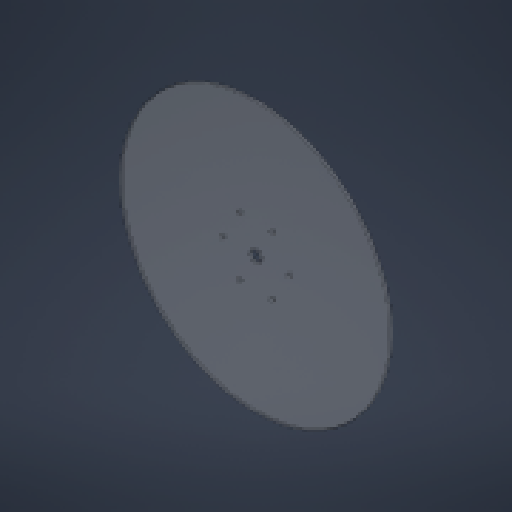
# Autodesk Inventor part: PLATE,BOTTOM
Saved by Autodesk Inventor 2026 (Build 300175000, 175)
## iProperties
Created: 2026-02-06
Part Number: PLATE,BOTTOM
Material: Polycarbonate, Clear
Document SubType Name: Sheet Metal
Designer: littl
Density: 1.2 g/cm^3
Sheet Metal Rule: Default
Appearance: Polycarbonate - Clear
Author: littl
Autodesk Inventor part; units mm, degrees
ref_plane "YZ Plane" through (0, 0, 0) normal (1, 0, 0) x (0, 1, 0)
ref_plane "XZ Plane" through (0, 0, 0) normal (0, 1, 0) x (-1, 0, 0)
ref_plane "XY Plane" through (0, 0, 0) normal (0, 0, 1) x (1, 0, 0)
sketch "Sketch1" plane through (0, 0, 0) normal (0, 0, 1) x (1, 0, 0)
  circle A0 centre (0, 0) radius 177.8
  dimension "d0" = 355.6
  measures "d0" diameter of A0
extrude "Plate1" add sketch "Sketch1" along normal blind 3.175
sketch "Sketch2" plane through (0, 0, 3.175) normal (0, 0, 1) x (1, 0, 0)
  line L0 (3.7395, -6.477) -> (-3.7395, -6.477)
  line L1 (-3.7395, -6.477) -> (-7.479, 0)
  line L2 (-7.479, 0) -> (-3.7395, 6.477)
  line L3 (-3.7395, 6.477) -> (3.7395, 6.477)
  line L4 (3.7395, 6.477) -> (7.479, 0)
  line L5 (7.479, 0) -> (3.7395, -6.477)
  point P0 (0, 0)
  point P1 (0, 0)
  dimension "d2" = 12.954
  constraints: 12 end point, 1 coincident, 1 horizontal, 13 other
  measures "d2" distance between parallel lines of L3 L0
extrude "Cut1" cut sketch "Sketch2" against normal blind 3.175
sketch "Sketch3" plane through (0, 0, 3.175) normal (0, 0, 1) x (1, 0, 0)
  point P0 (0, 0)
  point P1 (-44.45, 0)
  point P2 (-22.225, -38.4948)
  point P3 (22.225, -38.4948)
  point P4 (44.45, 0)
  point P5 (22.225, 38.4948)
  point P6 (-22.225, 38.4948)
  dimension "d5" = 44.45
  dimension "d8" = 360
  constraints: 1 horizontal alignment, 7 other
  measures "d5" distance of point (-44.45, 0) point (0, 0)
hole "Hole1" at (-44.45, 0, 3.175) at (-22.225, -38.4948, 3.175) at (22.225, -38.4948, 3.175) at (44.45, 0, 3.175) at (22.225, 38.4948, 3.175) at (-22.225, 38.4948, 3.175) direction (0, 0, -1) diameter 4.9784 end through all clearance for "Flat Head Machine Screw (82)" size "#10" standard "Ansi Unified Screw Threads"
equation "\"d3\" = Thickness"
equation "\"d15\" = Thickness"
equation "\"d1\" = Thickness"
equation "\"BendRadius\" = Thickness"
equation "\"BendReliefWidth\" = Thickness"
equation "\"BendReliefDepth\" = 0.5 * Thickness"
equation "\"CornerReliefSize\" = 4 * Thickness"
equation "\"MinimumRemnant\" = 2 * Thickness"
equation "\"TransitionRadius\" = BendRadius"
equation "\"JacobiRadiusSize\" = BendRadius"
equation "\"GapSize\" = Thickness"
equation "\"Thickness\" = 3.175"
body "Solid1"
